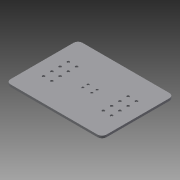
# Autodesk Inventor part: mic6_plate
Saved by Autodesk Inventor 2014 (Build 180170000, 170)
## iProperties
Created: 2014-08-09
Part Number: mic6_plate
Material: Generic
Document SubType Name: Modeling
Designer: Matthew
Density: 1 g/cm^3
Appearance: Default
Author: Matthew
Autodesk Inventor part; units mm, degrees
ref_plane "YZ Plane" through (0, 0, 0) normal (1, 0, 0) x (0, 1, 0)
ref_plane "XZ Plane" through (0, 0, 0) normal (0, 1, 0) x (-1, 0, 0)
ref_plane "XY Plane" through (0, 0, 0) normal (0, 0, 1) x (1, 0, 0)
sketch "Sketch1" plane through (0, 0, 0) normal (0, 1, 0) x (-1, 0, 0)
  line L0 (203.2, 152.4) -> (-203.2, 152.4)
  line L1 (-203.2, 152.4) -> (-203.2, -152.4)
  line L2 (-203.2, -152.4) -> (203.2, -152.4)
  line L3 (203.2, -152.4) -> (203.2, 152.4)
  line L4 (203.2, 152.4) -> (-203.2, -152.4) construction
  line L5 (-203.2, 152.4) -> (203.2, -152.4) construction
  point P0 (0, 0)
  dimension "d0" = 406.4
  dimension "d1" = 304.8
  constraints: 12 end point, 2 midpoint, 2 parallel, 1 horizontal, 1 perpendicular
  measures "d0" distance of L2.end L1.end
  measures "d1" distance of L0.end L1.end
extrude "Extrusion1" add sketch "Sketch1" along normal blind 9.525
fillet "Fillet1" radius 19.05 1 edges at (203.2, 4.7625, 152.4)
fillet "Fillet2" radius 19.05 1 edges at (203.2, 4.7625, -152.4)
fillet "Fillet3" radius 19.05 1 edges at (-203.2, 4.7625, 152.4)
fillet "Fillet4" radius 19.05 1 edges at (-203.2, 4.7625, -152.4)
sketch "Sketch2" plane through (0, 9.525, 0) normal (0, 1, 0) x (1, 0, 0)
  line L0 (-203.2, 133.35) -> (-203.2, -133.35) projected
  line L1 (-184.15, -152.4) -> (184.15, -152.4) projected
  point P0 (0, 0)
  point P1 (-177.8, -127)
  point P2 (-177.8, -76.2)
  point P3 (-177.8, -25.4)
  point P4 (-177.8, 25.4)
  point P5 (-177.8, 76.2)
  point P6 (-177.8, 127)
  point P7 (-152.4, -127)
  point P8 (-152.4, -76.2)
  point P9 (-152.4, -25.4)
  point P10 (-152.4, 25.4)
  point P11 (-152.4, 76.2)
  point P12 (-152.4, 127)
  point P13 (-127, -127)
  point P14 (-127, -76.2)
  point P15 (-127, -25.4)
  point P16 (-127, 25.4)
  point P17 (-127, 76.2)
  point P18 (-127, 127)
  point P19 (-101.6, -127)
  point P20 (-101.6, -76.2)
  point P21 (-101.6, -25.4)
  point P22 (-101.6, 25.4)
  point P23 (-101.6, 76.2)
  point P24 (-101.6, 127)
  point P25 (-76.2, -127)
  point P26 (-76.2, -76.2)
  point P27 (-76.2, -25.4)
  point P28 (-76.2, 25.4)
  point P29 (-76.2, 76.2)
  point P30 (-76.2, 127)
  point P31 (-50.8, -127)
  point P32 (-50.8, -76.2)
  point P33 (-50.8, -25.4)
  point P34 (-50.8, 25.4)
  point P35 (-50.8, 76.2)
  point P36 (-50.8, 127)
  point P37 (-25.4, -127)
  point P38 (-25.4, -76.2)
  point P39 (-25.4, -25.4)
  point P40 (-25.4, 25.4)
  point P41 (-25.4, 76.2)
  point P42 (-25.4, 127)
  point P43 (0, -127)
  point P44 (0, -76.2)
  point P45 (0, -25.4)
  point P46 (0, 25.4)
  point P47 (0, 76.2)
  point P48 (0, 127)
  point P49 (25.4, -127)
  point P50 (25.4, -76.2)
  point P51 (25.4, -25.4)
  point P52 (25.4, 25.4)
  point P53 (25.4, 76.2)
  point P54 (25.4, 127)
  point P55 (50.8, -127)
  point P56 (50.8, -76.2)
  point P57 (50.8, -25.4)
  point P58 (50.8, 25.4)
  point P59 (50.8, 76.2)
  point P60 (50.8, 127)
  point P61 (76.2, -127)
  point P62 (76.2, -76.2)
  point P63 (76.2, -25.4)
  point P64 (76.2, 25.4)
  point P65 (76.2, 76.2)
  point P66 (76.2, 127)
  dimension "d8" = 25.4
  dimension "d9" = 25.4
  dimension "d12" = 50.8
  dimension "d15" = 25.4
  constraints: 1 horizontal, 1 vertical, 65 other
  measures "d8" distance from line of point (-177.8, -127) L1
  measures "d9" distance from line of L0 point (-177.8, -127)
  measures "d12" distance of point (-177.8, -127) point (-177.8, -76.2)
  measures "d15" distance of point (-177.8, -127) point (-152.4, -127)
hole "Hole1" [suppressed]
sketch "Sketch3" plane through (0, 9.525, 0) normal (0, 1, 0) x (1, 0, 0)
  line L0 (-203.2, 133.35) -> (-203.2, -133.35) projected
  line L1 (184.15, 152.4) -> (-184.15, 152.4) projected
  line L2 (-150.5745, 60) -> (-150.5745, 10) construction
  line L3 (-150.5745, 10) -> (-102.5745, 10) construction
  line L4 (-102.5745, 10) -> (-102.5745, 60) construction
  line L5 (-102.5745, 60) -> (-150.5745, 60) construction
  line L6 (102.5745, 60) -> (102.5745, 10) construction
  line L7 (102.5745, 10) -> (150.5745, 10) construction
  line L8 (150.5745, 10) -> (150.5745, 60) construction
  line L9 (150.5745, 60) -> (102.5745, 60) construction
  line L10 (-150.5745, -10) -> (-150.5745, -60) construction
  line L11 (-150.5745, -60) -> (-102.5745, -60) construction
  line L12 (-102.5745, -60) -> (-102.5745, -10) construction
  line L13 (-102.5745, -10) -> (-150.5745, -10) construction
  line L14 (102.5745, -10) -> (102.5745, -60) construction
  line L15 (102.5745, -60) -> (150.5745, -60) construction
  line L16 (150.5745, -60) -> (150.5745, -10) construction
  line L17 (150.5745, -10) -> (102.5745, -10) construction
  line L18 (-24, 17.5) -> (24, 17.5) construction
  line L19 (24, 17.5) -> (24, -17.5) construction
  line L20 (24, -17.5) -> (-24, -17.5) construction
  line L21 (-24, -17.5) -> (-24, 17.5) construction
  line L22 (203.2, -133.35) -> (203.2, 133.35) projected
  point P0 (0, 0)
  point P1 (-144.0745, 52.5)
  point P2 (-109.0745, 52.5)
  point P3 (-144.0745, 17.5)
  point P4 (-109.0745, 17.5)
  point P5 (109.0745, 52.5)
  point P6 (144.0745, 52.5)
  point P7 (109.0745, 17.5)
  point P8 (144.0745, 17.5)
  point P9 (-144.0745, -17.5)
  point P10 (-109.0745, -17.5)
  point P11 (-144.0745, -52.5)
  point P12 (-109.0745, -52.5)
  point P13 (109.0745, -17.5)
  point P14 (144.0745, -17.5)
  point P15 (109.0745, -52.5)
  point P16 (144.0745, -52.5)
  point P17 (0, 17.5)
  point P18 (126.5745, 0)
  point P19 (24, 0)
  point P20 (126.5745, 60)
  point P21 (-19, 11)
  point P22 (19, 11)
  point P23 (-19, -11)
  point P24 (19, -11)
  dimension "d27" = 35
  dimension "d30" = 35
  dimension "d33" = 48
  dimension "d34" = 50
  dimension "d35" = 6.5
  dimension "d36" = 6.5
  dimension "d37" = 7.5
  dimension "d38" = 7.5
  dimension "d42" = 253.149
  dimension "d45" = 70
  dimension "d49" = 20
  dimension "d50" = 48
  dimension "d51" = 35
  dimension "d52" = 5
  dimension "d53" = 6.5
  dimension "d56" = 38
  dimension "d59" = 22
  dimension "d62" = 10
  dimension "d77" = 92.4
  dimension "d78" = 78.5745
  dimension "d79" = 78.5745
  dimension "d80" = 102.5745
  dimension "d109" = 48
  dimension "d110" = 52.6255
  constraints: 40 end point, 4 horizontal, 4 parallel, 3 midpoint, 3 perpendicular, 3 vertical, 2 horizontal alignment, 2 vertical alignment, 42 other
  measures "d27" distance of point (-144.075, 52.5) point (-109.074, 52.5)
  measures "d30" distance of point (-144.075, 52.5) point (-144.075, 17.5)
  measures "d33" distance of L2.end L3.end
  measures "d34" distance of L3.end L4.end
  measures "d35" distance from line of L4 point (-109.074, 52.5)
  measures "d36" distance from line of L2 point (-144.075, 52.5)
  measures "d37" distance from line of L5 point (-109.074, 52.5)
  measures "d38" distance from line of L3 point (-109.074, 17.5)
  measures "d42" distance of L2.start L6.start
  measures "d45" distance of L2.start L10.start
  measures "d49" distance between parallel lines of L3 L13
  measures "d50" distance of L19.end L20.end
  measures "d51" distance of L18.end L19.end
  measures "d52" distance from line of L21 point (-19, 11)
  measures "d53" distance from line of L18 point (-19, 11)
  measures "d56" distance of point (-19, 11) point (19, 11)
  measures "d59" distance of point (-19, 11) point (-19, -11)
  measures "d62" distance from line of L7 point (126.575, 0)
  measures "d77" distance between parallel lines of L1 L9
  measures "d78" distance between parallel lines of L21 L12
  measures "d79" distance between parallel lines of L14 L19
  measures "d80" horizontal distance of point (24, 0) point (126.575, 60)
  measures "d109" distance of L18.start L18.end
  measures "d110" distance between parallel lines of L22 L8
hole "Hole4" at (-144.0745, 9.525, -17.5) at (-144.0745, 9.525, -52.5) at (-109.0745, 9.525, -52.5) at (-109.0745, 9.525, 17.5) at (-109.0745, 9.525, -17.5) at (-144.0745, 9.525, 17.5) at (-144.0745, 9.525, 52.5) at (-109.0745, 9.525, 52.5) at (109.0745, 9.525, 17.5) at (144.0745, 9.525, 17.5) at (144.0745, 9.525, 52.5) at (109.0745, 9.525, 52.5) at (109.0745, 9.525, -52.5) at (144.0745, 9.525, -17.5) at (109.0745, 9.525, -17.5) at (144.0745, 9.525, -52.5) direction (0, -1, 0) diameter 5 depth 25.4 tip angle 118
hole "Hole5" at (-19, 9.525, -11) at (19, 9.525, -11) at (-19, 9.525, 11) at (19, 9.525, 11) direction (0, -1, 0) diameter 4 depth 25.4 tip angle 118
hole "Hole6" at (-144.0745, 9.525, -52.5) at (-109.0745, 9.525, -52.5) at (-109.0745, 9.525, -17.5) at (-144.0745, 9.525, -17.5) at (-144.0745, 9.525, 17.5) at (-109.0745, 9.525, 17.5) at (-109.0745, 9.525, 52.5) at (-144.0745, 9.525, 52.5) at (109.0745, 9.525, -52.5) at (144.0745, 9.525, -52.5) at (144.0745, 9.525, -17.5) at (109.0745, 9.525, -17.5) at (109.0745, 9.525, 17.5) at (144.0745, 9.525, 17.5) at (144.0745, 9.525, 52.5) at (109.0745, 9.525, 52.5) direction (0, -1, 0) diameter 11.2 depth 6
hole "Hole7" at (-19, 9.525, -11) at (19, 9.525, -11) at (19, 9.525, 11) at (-19, 9.525, 11) direction (0, -1, 0) diameter 9.75 depth 5
equation "\"d62\" = 0.5 * d49"
equation "\"d79\" = d78"
body "Solid1"
